Autodesk Fusion 360 part; units mm, degrees
(part 6 of 7)
extrude "Restore inletØ5 after outer sphere joins" cut sketch "Sketch35" along normal blind 11.45 contours A0 picked at (-21.937725, 164.26987) bodies 74 in component "Chamber / A3 top manifold with serial return"
ref_plane "WorkPlane36" through (0, 162.4, 0) normal (0, 1, 0) x (0, 0, 1) in component "Chamber / A3 top manifold with serial return"
sketch "Sketch36" plane through (0, 162.4, 0) normal (0, 1, 0) x (1, 0, 0) in component "Chamber / A3 top manifold with serial return"
  circle A0 centre (70.75, -22) radius 2.5
  dimension "d2207" = 70.75
  dimension "d2209" = 2.5
  measures "d2207" horizontal distance of origin A0.centre
  measures "d2209" radius of A0
extrude "Restore riseØ5 after outer sphere joins" cut sketch "Sketch36" along normal blind 2.7 contours A0 picked at (70.581043, -23.369363) bodies 74 in component "Chamber / A3 top manifold with serial return"
ref_plane "WorkPlane37" through (64.9, 0, 0) normal (1, 0, 0) x (0, 1, 0) in component "Chamber / A3 top manifold with serial return"
sketch "Sketch37" plane through (64.9, 0, 0) normal (1, 0, 0) x (0, 0, -1) in component "Chamber / A3 top manifold with serial return"
  circle A0 centre (-22, 165) radius 2.5
  dimension "d2215" = 165
  dimension "d2216" = 2.5
  measures "d2215" vertical distance of origin A0.centre
  measures "d2216" radius of A0
extrude "Restore exitØ5 through outer sphere into plenum" cut sketch "Sketch37" along normal blind 5.95 contours A0 picked at (-21.937725, 166.76987) bodies 74 in component "Chamber / A3 top manifold with serial return"
ref_plane "WorkPlane46" through (0, 0, 2.3) normal (0, 0, 1) x (1, 0, 0) in component "01 Shape A housing"
sketch "Cartridge front datum support sketch" plane through (0, 0, 2.3) normal (0, 0, 1) x (1, 0, 0) in component "01 Shape A housing"
  line L0 (6, 134) -> (12, 134)
  line L1 (12, 134) -> (12, 141)
  line L2 (12, 141) -> (6, 141)
  line L3 (6, 141) -> (6, 134)
  dimension "d2221" = 6
  dimension "d2222" = 134
  dimension "d2223" = 6
  dimension "d2224" = 7
  constraint horizontal L0
  constraint vertical L1
  constraint horizontal L2
  constraint vertical L3
  measures "d2221" horizontal distance of origin L0.start
  measures "d2222" vertical distance of origin L0.start
  measures "d2223" horizontal distance of L0.start L0.end
  measures "d2224" vertical distance of L0.end L1.end
extrude "Cartridge front datum support" add sketch "Cartridge front datum support sketch" along normal blind 0.7 contours L0 L1 L2 L3 picked at (10, 138.666667) bodies 1 in component "01 Shape A housing"
ref_plane "WorkPlane47" through (0, 0, 2.3) normal (0, 0, 1) x (1, 0, 0) in component "01 Shape A housing"
sketch "Cartridge front datum support sketch (1)" plane through (0, 0, 2.3) normal (0, 0, 1) x (1, 0, 0) in component "01 Shape A housing"
  line L0 (25, 152) -> (31, 152)
  line L1 (31, 152) -> (31, 159)
  line L2 (31, 159) -> (25, 159)
  line L3 (25, 159) -> (25, 152)
  dimension "d2229" = 25
  dimension "d2230" = 152
  dimension "d2231" = 6
  dimension "d2232" = 7
  constraint horizontal L0
  constraint vertical L1
  constraint horizontal L2
  constraint vertical L3
  measures "d2229" horizontal distance of origin L0.start
  measures "d2230" vertical distance of origin L0.start
  measures "d2231" horizontal distance of L0.start L0.end
  measures "d2232" vertical distance of L0.end L1.end
extrude "Cartridge front datum support (1)" add sketch "Cartridge front datum support sketch (1)" along normal blind 0.7 contours L0 L1 L2 L3 picked at (27, 156.666667) bodies 1 in component "01 Shape A housing"
ref_plane "WorkPlane48" through (0, 0, 2.3) normal (0, 0, 1) x (1, 0, 0) in component "01 Shape A housing"
sketch "Cartridge front datum support sketch (2)" plane through (0, 0, 2.3) normal (0, 0, 1) x (1, 0, 0) in component "01 Shape A housing"
  line L0 (53, 168) -> (60, 168)
  line L1 (60, 168) -> (60, 175)
  line L2 (60, 175) -> (53, 175)
  line L3 (53, 175) -> (53, 168)
  dimension "d2237" = 53
  dimension "d2238" = 168
  dimension "d2239" = 7
  dimension "d2240" = 7
  constraint horizontal L0
  constraint vertical L1
  constraint horizontal L2
  constraint vertical L3
  measures "d2237" horizontal distance of origin L0.start
  measures "d2238" vertical distance of origin L0.start
  measures "d2239" horizontal distance of L0.start L0.end
  measures "d2240" vertical distance of L0.end L1.end
extrude "Cartridge front datum support (2)" add sketch "Cartridge front datum support sketch (2)" along normal blind 0.7 contours L0 L1 L2 L3 picked at (55.333333, 172.666667) bodies 1 in component "01 Shape A housing"
ref_plane "WorkPlane49" through (0, 0, 2.3) normal (0, 0, 1) x (1, 0, 0) in component "01 Shape A housing"
sketch "Sketch49" plane through (0, 0, 2.3) normal (0, 0, 1) x (1, 0, 0) in component "01 Shape A housing"
  line L0 (25, 127.5) -> (35, 127.5)
  line L1 (35, 127.5) -> (35, 129.5)
  line L2 (35, 129.5) -> (25, 129.5)
  line L3 (25, 129.5) -> (25, 127.5)
  dimension "d2245" = 25
  dimension "d2246" = 127.5
  dimension "d2247" = 10
  dimension "d2248" = 2
  constraint horizontal L0
  constraint vertical L1
  constraint horizontal L2
  constraint vertical L3
  measures "d2245" horizontal distance of origin L0.start
  measures "d2246" vertical distance of origin L0.start
  measures "d2247" horizontal distance of L0.start L0.end
  measures "d2248" vertical distance of L0.end L1.end
extrude "Cartridge lower guide — clear harness exit" add sketch "Sketch49" along normal blind 35.5 contours L0 L1 L2 L3 picked at (28.333333, 128.833333) bodies 1 in component "01 Shape A housing"
ref_plane "WorkPlane50" through (0, 0, 2.3) normal (0, 0, 1) x (1, 0, 0) in component "01 Shape A housing"
sketch "Cartridge dry-side straight guide sketch" plane through (0, 0, 2.3) normal (0, 0, 1) x (1, 0, 0) in component "01 Shape A housing"
  line L0 (35.5, 130) -> (37.5, 130)
  line L1 (37.5, 130) -> (37.5, 132.1)
  line L2 (37.5, 132.1) -> (35.5, 132.1)
  line L3 (35.5, 132.1) -> (35.5, 130)
  dimension "d2253" = 35.5
  dimension "d2254" = 130
  dimension "d2255" = 2
  dimension "d2256" = 2.1
  constraint horizontal L0
  constraint vertical L1
  constraint horizontal L2
  constraint vertical L3
  measures "d2253" horizontal distance of origin L0.start
  measures "d2254" vertical distance of origin L0.start
  measures "d2255" horizontal distance of L0.start L0.end
  measures "d2256" vertical distance of L0.end L1.end
extrude "Cartridge dry-side straight guide" add sketch "Cartridge dry-side straight guide sketch" along normal blind 35.5 contours L0 L1 L2 L3 picked at (36.166667, 131.4) bodies 1 in component "01 Shape A housing"
ref_plane "WorkPlane51" through (0, 0, 2.3) normal (0, 0, 1) x (1, 0, 0) in component "01 Shape A housing"
sketch "Cartridge upper shoulder guide sketch" plane through (0, 0, 2.3) normal (0, 0, 1) x (1, 0, 0) in component "01 Shape A housing"
  line L0 (3.5, 167.5) -> (10.5, 167.5)
  line L1 (10.5, 167.5) -> (10.5, 169.5)
  line L2 (10.5, 169.5) -> (3.5, 169.5)
  line L3 (3.5, 169.5) -> (3.5, 167.5)
  dimension "d2261" = 3.5
  dimension "d2262" = 167.5
  dimension "d2263" = 7
  dimension "d2264" = 2
  constraint horizontal L0
  constraint vertical L1
  constraint horizontal L2
  constraint vertical L3
  measures "d2261" horizontal distance of origin L0.start
  measures "d2262" vertical distance of origin L0.start
  measures "d2263" horizontal distance of L0.start L0.end
  measures "d2264" vertical distance of L0.end L1.end
extrude "Cartridge upper shoulder guide" add sketch "Cartridge upper shoulder guide sketch" along normal blind 25.7 contours L0 L1 L2 L3 picked at (5.833333, 168.833333) bodies 1 in component "01 Shape A housing"
ref_plane "WorkPlane22" through (0, 0, 38.2) normal (0, 0, 1) x (1, 0, 0) in component "02 Single rear cover"
sketch "Closed cartridge rear capture stop sketch" plane through (0, 0, 38.2) normal (0, 0, 1) x (1, 0, 0) in component "02 Single rear cover"
  line L0 (6, 134) -> (12, 134)
  line L1 (12, 134) -> (12, 141)
  line L2 (12, 141) -> (6, 141)
  line L3 (6, 141) -> (6, 134)
  dimension "d2269" = 6
  dimension "d2270" = 134
  dimension "d2271" = 6
  dimension "d2272" = 7
  constraint horizontal L0
  constraint vertical L1
  constraint horizontal L2
  constraint vertical L3
  measures "d2269" horizontal distance of origin L0.start
  measures "d2270" vertical distance of origin L0.start
  measures "d2271" horizontal distance of L0.start L0.end
  measures "d2272" vertical distance of L0.end L1.end
extrude "Closed cartridge rear capture stop" add sketch "Closed cartridge rear capture stop sketch" along normal blind 2.7 contours L0 L1 L2 L3 picked at (10, 138.666667) bodies 4 in component "02 Single rear cover"
ref_plane "WorkPlane23" through (0, 0, 38.2) normal (0, 0, 1) x (1, 0, 0) in component "02 Single rear cover"
sketch "Closed cartridge rear capture stop sketch (1)" plane through (0, 0, 38.2) normal (0, 0, 1) x (1, 0, 0) in component "02 Single rear cover"
  line L0 (21, 150) -> (27, 150)
  line L1 (27, 150) -> (27, 156)
  line L2 (27, 156) -> (21, 156)
  line L3 (21, 156) -> (21, 150)
  dimension "d2277" = 21
  dimension "d2278" = 150
  dimension "d2279" = 6
  dimension "d2280" = 6
  constraint horizontal L0
  constraint vertical L1
  constraint horizontal L2
  constraint vertical L3
  measures "d2277" horizontal distance of origin L0.start
  measures "d2278" vertical distance of origin L0.start
  measures "d2279" horizontal distance of L0.start L0.end
  measures "d2280" vertical distance of L0.end L1.end
extrude "Closed cartridge rear capture stop (1)" add sketch "Closed cartridge rear capture stop sketch (1)" along normal blind 2.7 contours L0 L1 L2 L3 picked at (23, 154) bodies 4 in component "02 Single rear cover"
ref_plane "WorkPlane24" through (0, 0, 38.2) normal (0, 0, 1) x (1, 0, 0) in component "02 Single rear cover"
sketch "Closed cartridge rear capture stop sketch (2)" plane through (0, 0, 38.2) normal (0, 0, 1) x (1, 0, 0) in component "02 Single rear cover"
  line L0 (48, 166) -> (50, 166)
  line L1 (50, 166) -> (50, 173)
  line L2 (50, 173) -> (48, 173)
  line L3 (48, 173) -> (48, 166)
  dimension "d2285" = 48
  dimension "d2286" = 166
  dimension "d2287" = 2
  dimension "d2288" = 7
  constraint horizontal L0
  constraint vertical L1
  constraint horizontal L2
  constraint vertical L3
  measures "d2285" horizontal distance of origin L0.start
  measures "d2286" vertical distance of origin L0.start
  measures "d2287" horizontal distance of L0.start L0.end
  measures "d2288" vertical distance of L0.end L1.end
extrude "Closed cartridge rear capture stop (2)" add sketch "Closed cartridge rear capture stop sketch (2)" along normal blind 2.7 contours L0 L1 L2 L3 picked at (48.666667, 170.666667) bodies 4 in component "02 Single rear cover"
ref_plane "WorkPlane38" through (0, 0, 24.5) normal (0, 0, 1) x (1, 0, 0) in component "Chamber / A3 top manifold with serial return"
sketch "Provisional CO PCB left-face seat sketch" plane through (0, 0, 24.5) normal (0, 0, 1) x (1, 0, 0) in component "Chamber / A3 top manifold with serial return"
  line L0 (4.9, 133) -> (8.95, 133)
  line L1 (8.95, 133) -> (8.95, 135)
  line L2 (8.95, 135) -> (4.9, 135)
  line L3 (4.9, 135) -> (4.9, 133)
  dimension "d2293" = 4.9
  dimension "d2294" = 133
  dimension "d2295" = 4.05
  dimension "d2296" = 2
  constraint horizontal L0
  constraint vertical L1
  constraint horizontal L2
  constraint vertical L3
  measures "d2293" horizontal distance of origin L0.start
  measures "d2294" vertical distance of origin L0.start
  measures "d2295" horizontal distance of L0.start L0.end
  measures "d2296" vertical distance of L0.end L1.end
extrude "Provisional CO PCB left-face seat" add sketch "Provisional CO PCB left-face seat sketch" along normal blind 2 contours L0 L1 L2 L3 picked at (6.25, 134.333333) bodies 74 in component "Chamber / A3 top manifold with serial return"
ref_plane "WorkPlane39" through (0, 0, 8) normal (0, 0, 1) x (1, 0, 0) in component "Chamber / A3 top manifold with serial return"
sketch "Provisional CO PCB left-face seat sketch (1)" plane through (0, 0, 8) normal (0, 0, 1) x (1, 0, 0) in component "Chamber / A3 top manifold with serial return"
  line L0 (4.9, 155) -> (8.95, 155)
  line L1 (8.95, 155) -> (8.95, 157)
  line L2 (8.95, 157) -> (4.9, 157)
  line L3 (4.9, 157) -> (4.9, 155)
  dimension "d2301" = 4.9
  dimension "d2302" = 155
  dimension "d2303" = 4.05
  dimension "d2304" = 2
  constraint horizontal L0
  constraint vertical L1
  constraint horizontal L2
  constraint vertical L3
  measures "d2301" horizontal distance of origin L0.start
  measures "d2302" vertical distance of origin L0.start
  measures "d2303" horizontal distance of L0.start L0.end
  measures "d2304" vertical distance of L0.end L1.end
extrude "Provisional CO PCB left-face seat (1)" add sketch "Provisional CO PCB left-face seat sketch (1)" along normal blind 2 contours L0 L1 L2 L3 picked at (6.25, 156.333333) bodies 74 in component "Chamber / A3 top manifold with serial return"
ref_plane "WorkPlane40" through (0, 0, 4.9) normal (0, 0, 1) x (1, 0, 0) in component "Chamber / A3 top manifold with serial return"
sketch "Provisional CO front-edge seat sketch" plane through (0, 0, 4.9) normal (0, 0, 1) x (1, 0, 0) in component "Chamber / A3 top manifold with serial return"
  line L0 (8.75, 133) -> (10.75, 133)
  line L1 (10.75, 133) -> (10.75, 135)
  line L2 (10.75, 135) -> (8.75, 135)
  line L3 (8.75, 135) -> (8.75, 133)
  dimension "d2309" = 8.75
  dimension "d2310" = 133
  dimension "d2311" = 2
  dimension "d2312" = 2
  constraint horizontal L0
  constraint vertical L1
  constraint horizontal L2
  constraint vertical L3
  measures "d2309" horizontal distance of origin L0.start
  measures "d2310" vertical distance of origin L0.start
  measures "d2311" horizontal distance of L0.start L0.end
  measures "d2312" vertical distance of L0.end L1.end
extrude "Provisional CO front-edge seat" add sketch "Provisional CO front-edge seat sketch" along normal blind 0.5 contours L0 L1 L2 L3 picked at (9.416667, 134.333333) bodies 74 in component "Chamber / A3 top manifold with serial return"
ref_plane "WorkPlane41" through (0, 0, 6) normal (0, 0, 1) x (1, 0, 0) in component "Chamber / A3 top manifold with serial return"
sketch "Provisional CO upper corner keeper sketch" plane through (0, 0, 6) normal (0, 0, 1) x (1, 0, 0) in component "Chamber / A3 top manifold with serial return"
  line L0 (10.7, 155.5) -> (12.7, 155.5)
  line L1 (12.7, 155.5) -> (12.7, 159.5)
  line L2 (12.7, 159.5) -> (10.7, 159.5)
  line L3 (10.7, 159.5) -> (10.7, 155.5)
  dimension "d2317" = 10.7
  dimension "d2318" = 155.5
  dimension "d2319" = 2
  dimension "d2320" = 4
  constraint horizontal L0
  constraint vertical L1
  constraint horizontal L2
  constraint vertical L3
  measures "d2317" horizontal distance of origin L0.start
  measures "d2318" vertical distance of origin L0.start
  measures "d2319" horizontal distance of L0.start L0.end
  measures "d2320" vertical distance of L0.end L1.end
extrude "Provisional CO upper corner keeper" add sketch "Provisional CO upper corner keeper sketch" along normal blind 2 contours L0 L1 L2 L3 picked at (11.366667, 158.166667) bodies 74 in component "Chamber / A3 top manifold with serial return"
ref_plane "WorkPlane42" through (0, 0, 25) normal (0, 0, 1) x (1, 0, 0) in component "Chamber / A3 top manifold with serial return"
sketch "Provisional CO lower corner keeper sketch" plane through (0, 0, 25) normal (0, 0, 1) x (1, 0, 0) in component "Chamber / A3 top manifold with serial return"
  line L0 (10.7, 131.5) -> (12.7, 131.5)
  line L1 (12.7, 131.5) -> (12.7, 134.3)
  line L2 (12.7, 134.3) -> (10.7, 134.3)
  line L3 (10.7, 134.3) -> (10.7, 131.5)
  dimension "d2325" = 10.7
  dimension "d2326" = 131.5
  dimension "d2327" = 2
  dimension "d2328" = 2.8
  constraint horizontal L0
  constraint vertical L1
  constraint horizontal L2
  constraint vertical L3
  measures "d2325" horizontal distance of origin L0.start
  measures "d2326" vertical distance of origin L0.start
  measures "d2327" horizontal distance of L0.start L0.end
  measures "d2328" vertical distance of L0.end L1.end
extrude "Provisional CO lower corner keeper" add sketch "Provisional CO lower corner keeper sketch" along normal blind 2 contours L0 L1 L2 L3 picked at (11.366667, 133.366667) bodies 74 in component "Chamber / A3 top manifold with serial return"
ref_plane "WorkPlane43" through (0, 0, 4.9) normal (0, 0, 1) x (1, 0, 0) in component "Chamber / A3 top manifold with serial return"
sketch "Provisional MD62 front end-contact sketch" plane through (0, 0, 4.9) normal (0, 0, 1) x (1, 0, 0) in component "Chamber / A3 top manifold with serial return"
  line L0 (21.5, 164) -> (23.5, 164)
  line L1 (23.5, 164) -> (23.5, 166)
  line L2 (23.5, 166) -> (21.5, 166)
  line L3 (21.5, 166) -> (21.5, 164)
  dimension "d2333" = 21.5
  dimension "d2334" = 164
  dimension "d2335" = 2
  dimension "d2336" = 2
  constraint horizontal L0
  constraint vertical L1
  constraint horizontal L2
  constraint vertical L3
  measures "d2333" horizontal distance of origin L0.start
  measures "d2334" vertical distance of origin L0.start
  measures "d2335" horizontal distance of L0.start L0.end
  measures "d2336" vertical distance of L0.end L1.end
extrude "Provisional MD62 front end-contact" add sketch "Provisional MD62 front end-contact sketch" along normal blind 3.1 contours L0 L1 L2 L3 picked at (22.833333, 165.333333) bodies 74 in component "Chamber / A3 top manifold with serial return"
ref_plane "WorkPlane7" through (0, 0, 27.3) normal (0, 0, 1) x (1, 0, 0) in component "Chamber / A3 four-screw service lid"
sketch "Sketch7" plane through (0, 0, 27.3) normal (0, 0, 1) x (1, 0, 0) in component "Chamber / A3 four-screw service lid"
  line L0 (21.5, 164) -> (23.5, 164)
  line L1 (23.5, 164) -> (23.5, 166)
  line L2 (23.5, 166) -> (21.5, 166)
  line L3 (21.5, 166) -> (21.5, 164)
  dimension "d2341" = 21.5
  dimension "d2342" = 164
  dimension "d2343" = 2
  dimension "d2344" = 2
  constraint horizontal L0
  constraint vertical L1
  constraint horizontal L2
  constraint vertical L3
  measures "d2341" horizontal distance of origin L0.start
  measures "d2342" vertical distance of origin L0.start
  measures "d2343" horizontal distance of L0.start L0.end
  measures "d2344" vertical distance of L0.end L1.end
extrude "Provisional MD62 rear end-stop — 0.3 mm gap" add sketch "Sketch7" along normal blind 8.8 contours L0 L1 L2 L3 picked at (22.833333, 165.333333) bodies 75 in component "Chamber / A3 four-screw service lid"
ref_plane "WorkPlane44" through (0, 0, 4.9) normal (0, 0, 1) x (1, 0, 0) in component "Chamber / A3 top manifold with serial return"
sketch "Provisional MD62 front end-contact sketch (1)" plane through (0, 0, 4.9) normal (0, 0, 1) x (1, 0, 0) in component "Chamber / A3 top manifold with serial return"
  line L0 (21.5, 169.8) -> (23.5, 169.8)
  line L1 (23.5, 169.8) -> (23.5, 171.8)
  line L2 (23.5, 171.8) -> (21.5, 171.8)
  line L3 (21.5, 171.8) -> (21.5, 169.8)
  dimension "d2349" = 21.5
  dimension "d2350" = 169.8
  dimension "d2351" = 2
  dimension "d2352" = 2
  constraint horizontal L0
  constraint vertical L1
  constraint horizontal L2
  constraint vertical L3
  measures "d2349" horizontal distance of origin L0.start
  measures "d2350" vertical distance of origin L0.start
  measures "d2351" horizontal distance of L0.start L0.end
  measures "d2352" vertical distance of L0.end L1.end
extrude "Provisional MD62 front end-contact (1)" add sketch "Provisional MD62 front end-contact sketch (1)" along normal blind 3.1 contours L0 L1 L2 L3 picked at (22.166667, 171.133333) bodies 74 in component "Chamber / A3 top manifold with serial return"
ref_plane "WorkPlane8" through (0, 0, 27.3) normal (0, 0, 1) x (1, 0, 0) in component "Chamber / A3 four-screw service lid"
sketch "Sketch8" plane through (0, 0, 27.3) normal (0, 0, 1) x (1, 0, 0) in component "Chamber / A3 four-screw service lid"
  line L0 (21.5, 169.8) -> (23.5, 169.8)
  line L1 (23.5, 169.8) -> (23.5, 171.8)
  line L2 (23.5, 171.8) -> (21.5, 171.8)
  line L3 (21.5, 171.8) -> (21.5, 169.8)
  dimension "d2357" = 21.5
  dimension "d2358" = 169.8
  dimension "d2359" = 2
  dimension "d2360" = 2
  constraint horizontal L0
  constraint vertical L1
  constraint horizontal L2
  constraint vertical L3
  measures "d2357" horizontal distance of origin L0.start
  measures "d2358" vertical distance of origin L0.start
  measures "d2359" horizontal distance of L0.start L0.end
  measures "d2360" vertical distance of L0.end L1.end
extrude "Provisional MD62 rear end-stop — 0.3 mm gap (1)" add sketch "Sketch8" along normal blind 8.8 contours L0 L1 L2 L3 picked at (22.166667, 171.133333) bodies 75 in component "Chamber / A3 four-screw service lid"
ref_plane "WorkPlane45" through (0, 0, 4.9) normal (0, 0, 1) x (1, 0, 0) in component "Chamber / A3 top manifold with serial return"
sketch "Provisional MD62 lateral guide sketch" plane through (0, 0, 4.9) normal (0, 0, 1) x (1, 0, 0) in component "Chamber / A3 top manifold with serial return"
  line L0 (16.7, 163.5) -> (18.7, 163.5)
  line L1 (18.7, 163.5) -> (18.7, 171.5)
  line L2 (18.7, 171.5) -> (16.7, 171.5)
  line L3 (16.7, 171.5) -> (16.7, 163.5)
  dimension "d2365" = 16.7
  dimension "d2366" = 163.5
  dimension "d2367" = 2
  dimension "d2368" = 8
  constraint horizontal L0
  constraint vertical L1
  constraint horizontal L2
  constraint vertical L3
  measures "d2365" horizontal distance of origin L0.start
  measures "d2366" vertical distance of origin L0.start
  measures "d2367" horizontal distance of L0.start L0.end
  measures "d2368" vertical distance of L0.end L1.end
extrude "Provisional MD62 lateral guide" add sketch "Provisional MD62 lateral guide sketch" along normal blind 5.1 contours L0 L1 L2 L3 picked at (17.366667, 168.833333) bodies 74 in component "Chamber / A3 top manifold with serial return"
ref_plane "WorkPlane46" through (0, 0, 4.9) normal (0, 0, 1) x (1, 0, 0) in component "Chamber / A3 top manifold with serial return"
sketch "Provisional MD62 lateral guide sketch (1)" plane through (0, 0, 4.9) normal (0, 0, 1) x (1, 0, 0) in component "Chamber / A3 top manifold with serial return"
  line L0 (33.3, 163.5) -> (35.3, 163.5)
  line L1 (35.3, 163.5) -> (35.3, 171.5)
  line L2 (35.3, 171.5) -> (33.3, 171.5)
  line L3 (33.3, 171.5) -> (33.3, 163.5)
  dimension "d2373" = 33.3
  dimension "d2374" = 163.5
  dimension "d2375" = 2
  dimension "d2376" = 8
  constraint horizontal L0
  constraint vertical L1
  constraint horizontal L2
  constraint vertical L3
  measures "d2373" horizontal distance of origin L0.start
  measures "d2374" vertical distance of origin L0.start
  measures "d2375" horizontal distance of L0.start L0.end
  measures "d2376" vertical distance of L0.end L1.end
extrude "Provisional MD62 lateral guide (1)" add sketch "Provisional MD62 lateral guide sketch (1)" along normal blind 5.1 contours L0 L1 L2 L3 picked at (33.966667, 168.833333) bodies 74 in component "Chamber / A3 top manifold with serial return"
ref_plane "WorkPlane47" through (0, 0, 4.9) normal (0, 0, 1) x (1, 0, 0) in component "Chamber / A3 top manifold with serial return"
sketch "Provisional humidity PCB foot sketch" plane through (0, 0, 4.9) normal (0, 0, 1) x (1, 0, 0) in component "Chamber / A3 top manifold with serial return"
  line L0 (54, 164) -> (56, 164)
  line L1 (56, 164) -> (56, 166)
  line L2 (56, 166) -> (54, 166)
  line L3 (54, 166) -> (54, 164)
  dimension "d2381" = 54
  dimension "d2382" = 164
  dimension "d2383" = 2
  dimension "d2384" = 2
  constraint horizontal L0
  constraint vertical L1
  constraint horizontal L2
  constraint vertical L3
  measures "d2381" horizontal distance of origin L0.start
  measures "d2382" vertical distance of origin L0.start
  measures "d2383" horizontal distance of L0.start L0.end
  measures "d2384" vertical distance of L0.end L1.end
extrude "Provisional humidity PCB foot" add sketch "Provisional humidity PCB foot sketch" along normal blind 1.1 contours L0 L1 L2 L3 picked at (55.333333, 165.333333) bodies 74 in component "Chamber / A3 top manifold with serial return"
ref_plane "WorkPlane48" through (0, 0, 4.9) normal (0, 0, 1) x (1, 0, 0) in component "Chamber / A3 top manifold with serial return"
sketch "Provisional humidity PCB foot sketch (1)" plane through (0, 0, 4.9) normal (0, 0, 1) x (1, 0, 0) in component "Chamber / A3 top manifold with serial return"
  line L0 (67, 172) -> (69, 172)
  line L1 (69, 172) -> (69, 174)
  line L2 (69, 174) -> (67, 174)
  line L3 (67, 174) -> (67, 172)
  dimension "d2389" = 67
  dimension "d2390" = 172
  dimension "d2391" = 2
  dimension "d2392" = 2
  constraint horizontal L0
  constraint vertical L1
  constraint horizontal L2
  constraint vertical L3
  measures "d2389" horizontal distance of origin L0.start
  measures "d2390" vertical distance of origin L0.start
  measures "d2391" horizontal distance of L0.start L0.end
  measures "d2392" vertical distance of L0.end L1.end
extrude "Provisional humidity PCB foot (1)" add sketch "Provisional humidity PCB foot sketch (1)" along normal blind 1.1 contours L0 L1 L2 L3 picked at (67.666667, 173.333333) bodies 74 in component "Chamber / A3 top manifold with serial return"
ref_plane "WorkPlane49" through (0, 0, 7.9) normal (0, 0, 1) x (1, 0, 0) in component "Chamber / A3 top manifold with serial return"
sketch "Provisional humidity corner keeper sketch" plane through (0, 0, 7.9) normal (0, 0, 1) x (1, 0, 0) in component "Chamber / A3 top manifold with serial return"
  line L0 (68, 164) -> (70.6, 164)
  line L1 (70.6, 164) -> (70.6, 166)
  line L2 (70.6, 166) -> (68, 166)
  line L3 (68, 166) -> (68, 164)
  dimension "d2397" = 68
  dimension "d2398" = 164
  dimension "d2399" = 2.6
  dimension "d2400" = 2
  constraint horizontal L0
  constraint vertical L1
  constraint horizontal L2
  constraint vertical L3
  measures "d2397" horizontal distance of origin L0.start
  measures "d2398" vertical distance of origin L0.start
  measures "d2399" horizontal distance of L0.start L0.end
  measures "d2400" vertical distance of L0.end L1.end
extrude "Provisional humidity corner keeper" add sketch "Provisional humidity corner keeper sketch" along normal blind 2 contours L0 L1 L2 L3 picked at (69.733333, 165.333333) bodies 74 in component "Chamber / A3 top manifold with serial return"
ref_plane "WorkPlane9" through (0, -0.05, 0) normal (0, 1, 0) x (0, 0, 1) in component "USB A3 — tiny flush metal bezel and hidden flange"
sketch "PrintReview clean printable USB clearance throat rectangular stock sketch" plane through (0, -0.05, 0) normal (0, 1, 0) x (1, 0, 0) in component "USB A3 — tiny flush metal bezel and hidden flange"
  line L0 (37.55, -28.05) -> (47.45, -28.05)
  line L1 (47.45, -28.05) -> (47.45, -23.95)
  line L2 (47.45, -23.95) -> (37.55, -23.95)
  line L3 (37.55, -23.95) -> (37.55, -28.05)
  dimension "d2405" = 37.55
  dimension "d2406" = 28.05
  dimension "d2407" = 9.9
  dimension "d2408" = 4.1
  constraint horizontal L0
  constraint vertical L1
  constraint horizontal L2
  constraint vertical L3
  measures "d2405" horizontal distance of origin L0.start
  measures "d2406" vertical distance of origin L0.start
  measures "d2407" horizontal distance of L0.start L0.end
  measures "d2408" vertical distance of L0.end L1.end
extrude "PrintReview clean printable USB clearance throat rectangular stock" add sketch "PrintReview clean printable USB clearance throat rectangular stock sketch" along normal blind 1.9 separate body contours L0 L1 L2 L3 picked at (40.85, -25.316667) makes body 94 in component "USB A3 — tiny flush metal bezel and hidden flange"
fillet "PrintReview clean printable USB clearance throat corner rounds" radius 1.6 4 edges at (37.55, 0.9, 23.95) (47.45, 0.9, 23.95) (47.45, 0.9, 28.05) (37.55, 0.9, 28.05) on bodies 94 in component "USB A3 — tiny flush metal bezel and hidden flange"
combine "PrintReview clean printable USB clearance throat" operation cut target body 40 tool bodies 94 in component "USB A3 — tiny flush metal bezel and hidden flange"
ref_plane "WorkPlane9" through (0, 0, 32) normal (0, 0, 1) x (1, 0, 0) in component "USB A3 — hidden metal retaining bridge"
sketch "PrintReview PETG capture lip reinforcement sketch" plane through (0, 0, 32) normal (0, 0, 1) x (1, 0, 0) in component "USB A3 — hidden metal retaining bridge"
  line L0 (32.5, 3.6) -> (52.5, 3.6)
  line L1 (52.5, 3.6) -> (52.5, 6.4)
  line L2 (52.5, 6.4) -> (32.5, 6.4)
  line L3 (32.5, 6.4) -> (32.5, 3.6)
  dimension "d2415" = 32.5
  dimension "d2416" = 3.6
  dimension "d2417" = 20
  dimension "d2418" = 2.8
  constraint horizontal L0
  constraint vertical L1
  constraint horizontal L2
  constraint vertical L3
  measures "d2415" horizontal distance of origin L0.start
  measures "d2416" vertical distance of origin L0.start
  measures "d2417" horizontal distance of L0.start L0.end
  measures "d2418" vertical distance of L0.end L1.end
extrude "PrintReview PETG capture lip reinforcement" add sketch "PrintReview PETG capture lip reinforcement sketch" along normal blind 2 contours L0 L1 L2 L3 picked at (45.833333, 5.466667) bodies 48 in component "USB A3 — hidden metal retaining bridge"
thread "PrintReview modeled M16x1-6H female thread" "ISO Metric profile 16.0 M16x1 M16x1 6H" major diameter 16.1522 minor diameter 15.0355 pitch 1 angle 60 modelled right hand crest width 0.271947 on face at (37.533333, 140.895016, 29.689397) crest through (35.25, 142.5, 14.23225) on bodies 76 in component "Chamber / AO2 hand-tight adapter reference"
thread "AO2 nominal modeled mating thread; supplier fit unverified" "ISO Metric profile 16.0 M16x1 M16x1 6g" major diameter 15.884 minor diameter 14.741 pitch 1 angle 60 modelled right hand crest width 0.142909 on face at (36.833333, 141.703457, 13.789754) from (32.5, 142.5, 21.75) to (38.8, 142.5, 21.75) crest through (32.25, 142.5, 13.808) on bodies 77 in component "Sensor / AO2 dry body with wetted threaded nose"
ref_plane "WorkPlane50" through (0, 0, 33.5) normal (0, 0, 1) x (1, 0, 0) in component "Chamber / A3 top manifold with serial return"
sketch "PrintReview rear return open to removable lid sketch" plane through (0, 0, 33.5) normal (0, 0, 1) x (1, 0, 0) in component "Chamber / A3 top manifold with serial return"
  line L0 (5, 145.4) -> (10, 145.4)
  line L1 (10, 145.4) -> (10, 162.6)
  line L2 (10, 162.6) -> (5, 162.6)
  line L3 (5, 162.6) -> (5, 145.4)
  dimension "d2427" = 5
  dimension "d2428" = 145.4
  dimension "d2429" = 5
  dimension "d2430" = 17.2
  constraint horizontal L0
  constraint vertical L1
  constraint horizontal L2
  constraint vertical L3
  measures "d2427" horizontal distance of origin L0.start
  measures "d2428" vertical distance of origin L0.start
  measures "d2429" horizontal distance of L0.start L0.end
  measures "d2430" vertical distance of L0.end L1.end
extrude "PrintReview rear return open to removable lid" cut sketch "PrintReview rear return open to removable lid sketch" along normal blind 2.6 contours L0 L1 L2 L3 picked at (6.666667, 156.866667) bodies 74 in component "Chamber / A3 top manifold with serial return"
ref_plane "WorkPlane51" through (70.75, 0, 0) normal (1, 0, 0) x (0, 1, 0) in component "Chamber / A3 top manifold with serial return"
sketch "PrintReview main inlet outer support roof sketch" plane through (70.75, 0, 0) normal (1, 0, 0) x (0, 0, -1) in component "Chamber / A3 top manifold with serial return"
  line L0 (-25.181981, 159.318019) -> (-25.181981, 165.681981)
  line L1 (-25.181981, 165.681981) -> (-28.363961, 162.5)
  line L2 (-28.363961, 162.5) -> (-25.181981, 159.318019)
  dimension "d2435" = 25.181981
  dimension "d2436" = 159.318019
  dimension "d2437" = 25.181981
  dimension "d2438" = 165.681981
  dimension "d2439" = 28.363961
  dimension "d2440" = 162.5
extrude "PrintReview main inlet outer support roof" add sketch "PrintReview main inlet outer support roof sketch" along normal blind 11.25 contours L0 L1 L2 picked at (-26.242641, 162.5) bodies 74 in component "Chamber / A3 top manifold with serial return"
ref_plane "WorkPlane52" through (0, 162.5, 0) normal (0, 1, 0) x (0, 0, 1) in component "Chamber / A3 top manifold with serial return"
sketch "PrintReview inlet rise outer support roof sketch" plane through (0, 162.5, 0) normal (0, 1, 0) x (1, 0, 0) in component "Chamber / A3 top manifold with serial return"
  line L0 (67.568019, -25.181981) -> (73.931981, -25.181981)
  line L1 (73.931981, -25.181981) -> (70.75, -28.363961)
  line L2 (70.75, -28.363961) -> (67.568019, -25.181981)
  dimension "d2445" = 67.568019
  dimension "d2446" = 25.181981
  dimension "d2447" = 73.931981
  dimension "d2448" = 25.181981
  dimension "d2449" = 70.75
  dimension "d2450" = 28.363961
extrude "PrintReview inlet rise outer support roof" add sketch "PrintReview inlet rise outer support roof sketch" along normal blind 2.5 contours L0 L1 L2 picked at (70.75, -26.242641) bodies 74 in component "Chamber / A3 top manifold with serial return"
ref_plane "WorkPlane53" through (64.9, 0, 0) normal (1, 0, 0) x (0, 1, 0) in component "Chamber / A3 top manifold with serial return"
sketch "PrintReview upper turn outer support roof sketch" plane through (64.9, 0, 0) normal (1, 0, 0) x (0, 0, -1) in component "Chamber / A3 top manifold with serial return"
  line L0 (-25.181981, 161.818019) -> (-25.181981, 168.181981)
  line L1 (-25.181981, 168.181981) -> (-28.363961, 165)
  line L2 (-28.363961, 165) -> (-25.181981, 161.818019)
  dimension "d2455" = 25.181981
  dimension "d2456" = 161.818019
  dimension "d2457" = 25.181981
  dimension "d2458" = 168.181981
  dimension "d2459" = 28.363961
  dimension "d2460" = 165
extrude "PrintReview upper turn outer support roof" add sketch "PrintReview upper turn outer support roof sketch" along normal blind 5.85 contours L0 L1 L2 picked at (-26.242641, 165) bodies 74 in component "Chamber / A3 top manifold with serial return"
ref_plane "WorkPlane54" through (0, 0, 25.171981) normal (0, 0, 1) x (1, 0, 0) in component "Chamber / A3 top manifold with serial return"
sketch "PrintReview elbow outer self-support roof base" plane through (0, 0, 25.171981) normal (0, 0, 1) x (1, 0, 0) in component "Chamber / A3 top manifold with serial return"
  circle A0 centre (70.75, 162.5) radius 3.191981
  dimension "d2465" = 70.75
  dimension "d2466" = 162.5
  dimension "d2467" = 3.191981
  measures "d2465" horizontal distance of origin A0.centre
  measures "d2466" vertical distance of origin A0.centre
  measures "d2467" radius of A0
ref_plane "WorkPlane55" through (0, 0, 28.313961) normal (0, 0, 1) x (1, 0, 0) in component "Chamber / A3 top manifold with serial return"
sketch "PrintReview elbow outer self-support roof tiny printable crest" plane through (0, 0, 28.313961) normal (0, 0, 1) x (1, 0, 0) in component "Chamber / A3 top manifold with serial return"
  circle A0 centre (70.75, 162.5) radius 0.05
  dimension "d2470" = 70.75
  dimension "d2471" = 162.5
  dimension "d2472" = 0.05
  measures "d2470" horizontal distance of origin A0.centre
  measures "d2471" vertical distance of origin A0.centre
  measures "d2472" radius of A0
loft "PrintReview elbow outer self-support roof" add profiles "PrintReview elbow outer self-support roof base", "PrintReview elbow outer self-support roof tiny printable crest" section 1 contours A0 picked at (71.413389, 163.959099) section 2 contours A0 picked at (70.734984, 162.507231) bodies 74 in component "Chamber / A3 top manifold with serial return"
ref_plane "WorkPlane56" through (0, 0, 25.171981) normal (0, 0, 1) x (1, 0, 0) in component "Chamber / A3 top manifold with serial return"
sketch "PrintReview elbow outer self-support roof base (1)" plane through (0, 0, 25.171981) normal (0, 0, 1) x (1, 0, 0) in component "Chamber / A3 top manifold with serial return"
  circle A0 centre (70.75, 165) radius 3.191981
  dimension "d2475" = 70.75
  dimension "d2476" = 165
  dimension "d2477" = 3.191981
  measures "d2475" horizontal distance of origin A0.centre
  measures "d2476" vertical distance of origin A0.centre
  measures "d2477" radius of A0
ref_plane "WorkPlane57" through (0, 0, 28.313961) normal (0, 0, 1) x (1, 0, 0) in component "Chamber / A3 top manifold with serial return"
sketch "PrintReview elbow outer self-support roof tiny printable crest (1)" plane through (0, 0, 28.313961) normal (0, 0, 1) x (1, 0, 0) in component "Chamber / A3 top manifold with serial return"
  circle A0 centre (70.75, 165) radius 0.05
  dimension "d2480" = 70.75
  dimension "d2481" = 165
  dimension "d2482" = 0.05
  measures "d2480" horizontal distance of origin A0.centre
  measures "d2481" vertical distance of origin A0.centre
  measures "d2482" radius of A0
loft "PrintReview elbow outer self-support roof (1)" add profiles "PrintReview elbow outer self-support roof base (1)", "PrintReview elbow outer self-support roof tiny printable crest (1)" section 1 contours A0 picked at (71.413389, 166.459099) section 2 contours A0 picked at (70.734984, 165.007231) bodies 74 in component "Chamber / A3 top manifold with serial return"
ref_plane "WorkPlane58" through (70.75, 0, 0) normal (1, 0, 0) x (0, 1, 0) in component "Chamber / A3 top manifold with serial return"
sketch "PrintReview main inlet internal 45 degree roof sketch" plane through (70.75, 0, 0) normal (1, 0, 0) x (0, 0, -1) in component "Chamber / A3 top manifold with serial return"
  line L0 (-23.767767, 160.732233) -> (-23.767767, 164.267767)
  line L1 (-23.767767, 164.267767) -> (-25.535534, 162.5)
  line L2 (-25.535534, 162.5) -> (-23.767767, 160.732233)
  dimension "d2485" = 23.767767
  dimension "d2486" = 160.732233
  dimension "d2487" = 23.767767
  dimension "d2488" = 164.267767
  dimension "d2489" = 25.535534
  dimension "d2490" = 162.5
extrude "PrintReview main inlet internal 45 degree roof" cut sketch "PrintReview main inlet internal 45 degree roof sketch" along normal blind 11.25 contours L0 L1 L2 picked at (-24.357023, 162.5) bodies 74 in component "Chamber / A3 top manifold with serial return"
ref_plane "WorkPlane59" through (0, 162.5, 0) normal (0, 1, 0) x (0, 0, 1) in component "Chamber / A3 top manifold with serial return"
sketch "PrintReview inlet rise internal 45 degree roof sketch" plane through (0, 162.5, 0) normal (0, 1, 0) x (1, 0, 0) in component "Chamber / A3 top manifold with serial return"
  line L0 (68.982233, -23.767767) -> (72.517767, -23.767767)
  line L1 (72.517767, -23.767767) -> (70.75, -25.535534)
  line L2 (70.75, -25.535534) -> (68.982233, -23.767767)
  dimension "d2495" = 68.982233
  dimension "d2496" = 23.767767
  dimension "d2497" = 72.517767
  dimension "d2498" = 23.767767
  dimension "d2499" = 70.75
  dimension "d2500" = 25.535534
extrude "PrintReview inlet rise internal 45 degree roof" cut sketch "PrintReview inlet rise internal 45 degree roof sketch" along normal blind 2.5 contours L0 L1 L2 picked at (70.75, -24.357023) bodies 74 in component "Chamber / A3 top manifold with serial return"
ref_plane "WorkPlane60" through (64.9, 0, 0) normal (1, 0, 0) x (0, 1, 0) in component "Chamber / A3 top manifold with serial return"
sketch "PrintReview upper turn internal 45 degree roof sketch" plane through (64.9, 0, 0) normal (1, 0, 0) x (0, 0, -1) in component "Chamber / A3 top manifold with serial return"
  line L0 (-23.767767, 163.232233) -> (-23.767767, 166.767767)
  line L1 (-23.767767, 166.767767) -> (-25.535534, 165)
  line L2 (-25.535534, 165) -> (-23.767767, 163.232233)
  dimension "d2505" = 23.767767
  dimension "d2506" = 163.232233
  dimension "d2507" = 23.767767
  dimension "d2508" = 166.767767
  dimension "d2509" = 25.535534
  dimension "d2510" = 165
extrude "PrintReview upper turn internal 45 degree roof" cut sketch "PrintReview upper turn internal 45 degree roof sketch" along normal blind 5.85 contours L0 L1 L2 picked at (-24.357023, 165) bodies 74 in component "Chamber / A3 top manifold with serial return"
ref_plane "WorkPlane61" through (0, 0, 23.757767) normal (0, 0, 1) x (1, 0, 0) in component "Chamber / A3 top manifold with serial return"
sketch "PrintReview elbow internal self-support roof base" plane through (0, 0, 23.757767) normal (0, 0, 1) x (1, 0, 0) in component "Chamber / A3 top manifold with serial return"
  circle A0 centre (70.75, 162.5) radius 1.777767
  dimension "d2515" = 70.75
  dimension "d2516" = 162.5
  dimension "d2517" = 1.777767
  measures "d2515" horizontal distance of origin A0.centre
  measures "d2516" vertical distance of origin A0.centre
  measures "d2517" radius of A0
ref_plane "WorkPlane62" through (0, 0, 25.485534) normal (0, 0, 1) x (1, 0, 0) in component "Chamber / A3 top manifold with serial return"
sketch "PrintReview elbow internal self-support roof tiny printable crest" plane through (0, 0, 25.485534) normal (0, 0, 1) x (1, 0, 0) in component "Chamber / A3 top manifold with serial return"
  circle A0 centre (70.75, 162.5) radius 0.05
  dimension "d2520" = 70.75
  dimension "d2521" = 162.5
  dimension "d2522" = 0.05
  measures "d2520" horizontal distance of origin A0.centre
  measures "d2521" vertical distance of origin A0.centre
  measures "d2522" radius of A0
loft "PrintReview elbow internal self-support roof" cut profiles "PrintReview elbow internal self-support roof base", "PrintReview elbow internal self-support roof tiny printable crest" section 1 contours A0 picked at (70.453706, 161.472573) section 2 contours A0 picked at (70.734984, 162.507231) bodies 74 in component "Chamber / A3 top manifold with serial return"
ref_plane "WorkPlane63" through (0, 0, 23.757767) normal (0, 0, 1) x (1, 0, 0) in component "Chamber / A3 top manifold with serial return"
sketch "PrintReview elbow internal self-support roof base (1)" plane through (0, 0, 23.757767) normal (0, 0, 1) x (1, 0, 0) in component "Chamber / A3 top manifold with serial return"
  circle A0 centre (70.75, 165) radius 1.777767
  dimension "d2525" = 70.75
  dimension "d2526" = 165
  dimension "d2527" = 1.777767
  measures "d2525" horizontal distance of origin A0.centre
  measures "d2526" vertical distance of origin A0.centre
  measures "d2527" radius of A0
ref_plane "WorkPlane64" through (0, 0, 25.485534) normal (0, 0, 1) x (1, 0, 0) in component "Chamber / A3 top manifold with serial return"
sketch "PrintReview elbow internal self-support roof tiny printable crest (1)" plane through (0, 0, 25.485534) normal (0, 0, 1) x (1, 0, 0) in component "Chamber / A3 top manifold with serial return"
  circle A0 centre (70.75, 165) radius 0.05
  dimension "d2530" = 70.75
  dimension "d2531" = 165
  dimension "d2532" = 0.05
  measures "d2530" horizontal distance of origin A0.centre
  measures "d2531" vertical distance of origin A0.centre
  measures "d2532" radius of A0
loft "PrintReview elbow internal self-support roof (1)" cut profiles "PrintReview elbow internal self-support roof base (1)", "PrintReview elbow internal self-support roof tiny printable crest (1)" section 1 contours A0 picked at (70.453706, 163.972573) section 2 contours A0 picked at (70.734984, 165.007231) bodies 74 in component "Chamber / A3 top manifold with serial return"
ref_plane "WorkPlane65" through (2.9, 0, 0) normal (1, 0, 0) x (0, 1, 0) in component "Chamber / A3 top manifold with serial return"
sketch "PrintReview exhaust wall internal 45 degree roof sketch" plane through (2.9, 0, 0) normal (1, 0, 0) x (0, 0, -1) in component "Chamber / A3 top manifold with serial return"
  line L0 (-23.767767, 160.732233) -> (-23.767767, 164.267767)
  line L1 (-23.767767, 164.267767) -> (-25.535534, 162.5)
  line L2 (-25.535534, 162.5) -> (-23.767767, 160.732233)
  dimension "d2535" = 23.767767
  dimension "d2536" = 160.732233
  dimension "d2537" = 23.767767
  dimension "d2538" = 164.267767
  dimension "d2539" = 25.535534
  dimension "d2540" = 162.5
extrude "PrintReview exhaust wall internal 45 degree roof" cut sketch "PrintReview exhaust wall internal 45 degree roof sketch" along normal blind 4.7 contours L0 L1 L2 picked at (-24.357023, 162.5) bodies 74 in component "Chamber / A3 top manifold with serial return"
ref_plane "WorkPlane3" through (0, 0, 21.75) normal (0, 0, 1) x (1, 0, 0) in component "Sensor / AO2 dry body with wetted threaded nose"
sketch "AO2 rotation centreline" plane through (0, 0, 21.75) normal (0, 0, 1) x (1, 0, 0) in component "Sensor / AO2 dry body with wetted threaded nose"
  line L0 (0, 142.5) -> (10, 142.5)
  dimension "d2545" = 142.5
  dimension "d2546" = 10
  constraint vertical origin L0.start
  constraint horizontal L0
  measures "d2545" vertical distance of origin L0.start
  measures "d2546" horizontal distance of L0.start L0.end
move_body "AO2 nominal thread phase aligned for mating CAD" bodies 77 to x (1, 0, 0) y (0, -1, 0) z (0, 0, -1) at (0, 285, 43.5) in component "Sensor / AO2 dry body with wetted threaded nose"
chamfer "PrintReview four rear locating tab lead-ins 0.30mm" distance 0.3 angle 45 16 edges at (80.35, 104, 38.6) (81.35, 110, 38.6) (82.35, 104, 38.6) (81.35, 98, 38.6) (80.35, 61, 38.6) (81.35, 67, 38.6) (82.35, 61, 38.6) (81.35, 55, 38.6) (2.65, 104, 38.6) (3.65, 110, 38.6) (4.65, 104, 38.6) (3.65, 98, 38.6) (2.65, 61, 38.6) (3.65, 67, 38.6) (4.65, 61, 38.6) (3.65, 55, 38.6) tangent chain off on bodies 4 in component "02 Single rear cover"
component "01 Shape A housing" placed x (1, 0, 0) y (0, 1, 0) z (0, 0, 1) at (0, 0, 0)
component "02 Single rear cover" placed x (1, 0, 0) y (0, 1, 0) z (0, 0, 1) at (0, 0, 0)
component "M3 x 8 button screw — GEN-M3-BHCS-L8-AF2" placed x (1, 0, 0) y (0, 1, 0) z (0, 0, 1) at (8, 8, 41.35)
component "M3 insert OD4.2 x5 — GEN-M3-HEATSET-OD4.2-L5" placed x (1, 0, 0) y (0, 1, 0) z (0, 0, 1) at (8, 8, 39)
component "Carrier / removable electronics tray" placed x (1, 0, 0) y (0, 1, 0) z (0, 0, 1) at (0, 0, 0)
component "Carrier / future PCB allocation — layout pending" placed x (1, 0, 0) y (0, 1, 0) z (0, 0, 1) at (0, 0, 0)
component "M2 x 7 socket_cap screw — GEN-M2-SHCS-L7-AF1.5" placed x (1, 0, 0) y (0, 1, 0) z (0, 0, 1) at (76, 28, 22.1)
component "M2 insert OD3.2 x4 — GEN-M2-HEATSET-OD3.2-L4" placed x (1, 0, 0) y (0, 1, 0) z (0, 0, 1) at (76, 28, 18.5)
component "Display / lower rear-release retainer" placed x (1, 0, 0) y (0, 1, 0) z (0, 0, 1) at (0, 0, 0)
component "Display / upper rear-release retainer" placed x (1, 0, 0) y (0, 1, 0) z (0, 0, 1) at (0, 0, 0)
component "M2 x 5 socket_cap screw — GEN-M2-SHCS-L5-AF1.5" placed x (1, 0, 0) y (0, 1, 0) z (0, 0, 1) at (69, 12.3, 20.5)
component "Battery / FMA protected holder - owner-measured envelope" placed x (1, 0, 0) y (0, 1, 0) z (0, 0, 1) at (0, 0, 0)
component "Battery / 18650 cell A - owner-rated 3400 mAh" placed x (1, 0, 0) y (0, 1, 0) z (0, 0, 1) at (0, 0, 0)
component "Battery / 18650 cell B - owner-rated 3400 mAh" placed x (1, 0, 0) y (0, 1, 0) z (0, 0, 1) at (0, 0, 0)
component "Battery / red RCY disconnect body - provisional reference" placed x (1, 0, 0) y (0, 1, 0) z (0, 0, 1) at (0, 0, 0)
component "Battery / red RCY disconnect mate - provisional reference" placed x (1, 0, 0) y (0, 1, 0) z (0, 0, 1) at (0, 0, 0)
component "USB A3 — tiny flush metal bezel and hidden flange" placed x (1, 0, 0) y (0, 1, 0) z (0, 0, 1) at (0, 0, 0)
component "USB A3 — removable printed support frame" placed x (1, 0, 0) y (0, 1, 0) z (0, 0, 1) at (0, 0, 0)
component "USB A3 — hidden metal retaining bridge" placed x (1, 0, 0) y (0, 1, 0) z (0, 0, 1) at (0, 0, 0)
component "USB A3 — supported 0.60 mm daughterboard provisional" placed x (1, 0, 0) y (0, 1, 0) z (0, 0, 1) at (0, 0, 0)
component "Chamber / A3 top manifold with serial return" placed x (1, 0, 0) y (0, 1, 0) z (0, 0, 1) at (0, 0, 0)
component "Chamber / A3 four-screw service lid" placed x (1, 0, 0) y (0, 1, 0) z (0, 0, 1) at (0, 0, 0)
component "Chamber / AO2 hand-tight adapter reference" placed x (1, 0, 0) y (0, 1, 0) z (0, 0, 1) at (0, 0, 0)
component "Sensor / AO2 dry body with wetted threaded nose" placed x (1, 0, 0) y (0, 1, 0) z (0, 0, 1) at (0, 0, 0)
component "Sensor / AO2 cable connector allowance" placed x (1, 0, 0) y (0, 1, 0) z (0, 0, 1) at (0, 0, 0)
component "Sensor / ZE07-CO drawing-derived assembly" placed x (1, 0, 0) y (0, 1, 0) z (0, 0, 1) at (0, 0, 0)
component "Sensor / MD62 body and full-length lead references" placed x (1, 0, 0) y (0, 1, 0) z (0, 0, 1) at (0, 0, 0)
component "Sensor / GYBMEP humidity breakout reference" placed x (1, 0, 0) y (0, 1, 0) z (0, 0, 1) at (0, 0, 0)
component "Gas / Viewer-left inlet fitting reference" placed x (1, 0, 0) y (0, 1, 0) z (0, 0, 1) at (0, 0, 0)
component "Gas / Viewer-right exhaust fitting reference" placed x (1, 0, 0) y (0, 1, 0) z (0, 0, 1) at (0, 0, 0)
component "Chamber / AO2 face-seal allowance" placed x (1, 0, 0) y (0, 1, 0) z (0, 0, 1) at (0, 0, 0)
component "Chamber / sealed harness feedthrough allowance" placed x (1, 0, 0) y (0, 1, 0) z (0, 0, 1) at (0, 0, 0)
component "M3 x 8 button screw — GEN-M3-BHCS-L8-AF2" placed x (1, 0, 0) y (0, 1, 0) z (0, 0, 1) at (77, 8, 41.35)
component "M3 x 8 button screw — GEN-M3-BHCS-L8-AF2" placed x (1, 0, 0) y (0, 1, 0) z (0, 0, 1) at (8, 172, 41.35)
component "M3 x 8 button screw — GEN-M3-BHCS-L8-AF2" placed x (1, 0, 0) y (0, 1, 0) z (0, 0, 1) at (77, 172, 41.35)
component "M3 insert OD4.2 x5 — GEN-M3-HEATSET-OD4.2-L5" placed x (1, 0, 0) y (0, 1, 0) z (0, 0, 1) at (77, 8, 39)
component "M3 insert OD4.2 x5 — GEN-M3-HEATSET-OD4.2-L5" placed x (1, 0, 0) y (0, 1, 0) z (0, 0, 1) at (8, 172, 39)
component "M3 insert OD4.2 x5 — GEN-M3-HEATSET-OD4.2-L5" placed x (1, 0, 0) y (0, 1, 0) z (0, 0, 1) at (77, 172, 39)
component "M2 x 7 socket_cap screw — GEN-M2-SHCS-L7-AF1.5" placed x (1, 0, 0) y (0, 1, 0) z (0, 0, 1) at (54.8, 114, 22.1)